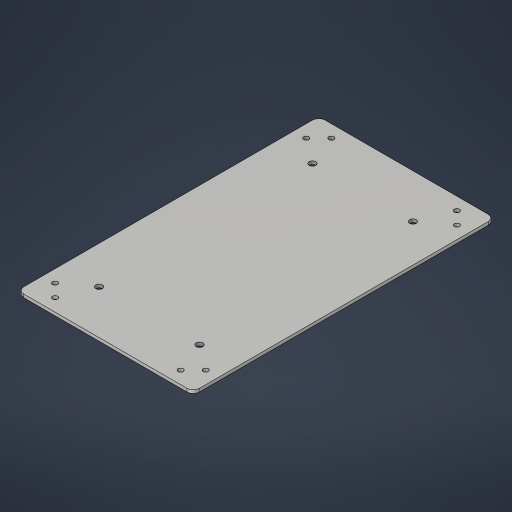
# Autodesk Inventor part: PDP_Plate
Saved by Autodesk Inventor 2023 (Build 270158000, 158)
## iProperties
Created: 2022-12-12
Part Number: PDP_Plate
Material: Aluminum 5052 H32
Document SubType Name: Sheet Metal
Designer: Conno
Mass: 461.668 g
Surface Area: 1114.14 cm^2
Volume: 170.988 cm^3
Density: 2.7 g/cm^3
Sheet Metal Rule: .125 5052
Appearance: Aluminum - Flat
Description: Plate to support the PDP
DocNumber: PDP_Plate.ipt
Folder: 2023\Swerve Electrical Concept\
VDS_Category: CAD
Author: Conno
Autodesk Inventor part; units mm, degrees
ref_plane "YZ Plane" through (0, 0, 0) normal (1, 0, 0) x (0, 1, 0)
ref_plane "XZ Plane" through (0, 0, 0) normal (0, 1, 0) x (-1, 0, 0)
ref_plane "XY Plane" through (0, 0, 0) normal (0, 0, 1) x (1, 0, 0)
sketch "Sketch1" plane through (0, 0, 0) normal (0, 1, 0) x (-1, 0, 0)
  line L0 (88.9, -152.4) -> (-88.9, -152.4)
  line L1 (-88.9, -152.4) -> (-88.9, 152.4)
  line L2 (-88.9, 152.4) -> (88.9, 152.4)
  line L3 (88.9, 152.4) -> (88.9, -152.4)
  line L4 (88.9, -152.4) -> (-88.9, 152.4) construction
  line L5 (-88.9, -152.4) -> (88.9, 152.4) construction
  point P0 (0, 0)
  dimension "d0" = 177.8
  dimension "d1" = 304.8
  measures "d0" distance of L1.end L2.end
  measures "d1" distance of L0.end L1.end
extrude "Plate1" add sketch "Sketch1" along normal blind 3.175
fillet "Corner Round1" radius 6.35 4 edges at (-88.9, 1.5875, 152.4) (88.9, 1.5875, 152.4) (-88.9, 1.5875, -152.4) (88.9, 1.5875, -152.4)
sketch "Sketch2" plane through (0, 3.175, 0) normal (0, 1, 0) x (1, 0, 0)
  circle A0 centre (-76.2, 127) radius 2.5797
  line L0 (-88.9, -146.05) -> (-88.9, 146.05) projected
  line L1 (-82.55, 152.4) -> (82.55, 152.4) projected
  circle A1 centre (-63.5, 139.7) radius 2.5797
  line L2 (-88.9, 0) -> (88.9, 0) construction
  line L3 (88.9, 146.05) -> (88.9, -146.05) construction
  line L4 (-82.55, 152.4) -> (82.55, 152.4) construction
  line L5 (0, 152.4) -> (0, -152.4) construction
  line L6 (82.55, -152.4) -> (-82.55, -152.4) construction
  circle A2 centre (76.2, 127) radius 2.5797
  circle A3 centre (63.5, 139.7) radius 2.5797
  circle A4 centre (-76.2, -127) radius 2.5797
  circle A5 centre (-63.5, -139.7) radius 2.5797
  circle A6 centre (63.5, -139.7) radius 2.5797
  circle A7 centre (76.2, -127) radius 2.5797
  circle A8 centre (-50.8, 107.95) radius 3.302
  line L7 (-50.8, 107.95) -> (50.8, 107.95) construction
  circle A9 centre (50.8, 107.95) radius 3.302
  line L8 (50.8, 107.95) -> (50.8, -107.95) construction
  circle A10 centre (50.8, -107.95) radius 3.302
  line L9 (50.8, -107.95) -> (-50.8, -107.95) construction
  circle A11 centre (-50.8, -107.95) radius 3.302
  line L10 (-50.8, 107.95) -> (-50.8, -107.95) construction
  point P0 (0, 0)
  point P1 (0, 107.95)
  point P2 (-50.8, 0)
  dimension "d4" = 5.1594
  dimension "d5" = 12.7
  dimension "d6" = 25.4
  dimension "d7" = 12.7
  dimension "d8" = 25.4
  dimension "d11" = 101.6
  dimension "d12" = 6.604
  dimension "d13" = 215.9
  constraints: 12 centre point, 12 end point, 6 midpoint, 6 symmetric about line, 4 equal radius, 3 coincident, 2 horizontal, 2 point on line, 1 parallel, 1 perpendicular, 1 vertical, 6 other
  measures "d4" diameter of A0
  measures "d5" distance from line of L0 A0.centre
  measures "d6" distance from line of L1 A0.centre
  measures "d7" distance from line of L1 A1.centre
  measures "d8" distance from line of L0 A1.centre
  measures "d11" distance of L7.start L7.end
  measures "d12" diameter of A9
  measures "d13" distance of L8.start L8.end
extrude "Cut1" cut sketch "Sketch2" against normal blind 3.175
equation "\"d9\" = Thickness"
equation "\"d2\" = Thickness"
equation "\"BendRadius\" = 1.5 * Thickness"
equation "\"BendReliefWidth\" = Thickness"
equation "\"BendReliefDepth\" = 0.5 * Thickness"
equation "\"CornerReliefSize\" = 4 * Thickness"
equation "\"MinimumRemnant\" = 2 * Thickness"
equation "\"TransitionRadius\" = BendRadius"
equation "\"JacobiRadiusSize\" = BendRadius"
equation "\"GapSize\" = Thickness"
equation "\"Thickness\" = 3.175"
body "Solid1"
